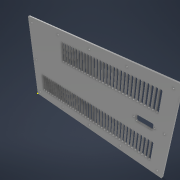
# Autodesk Inventor part: BackShield
Saved by Autodesk Inventor 2022 (Build 260153000, 153)
## iProperties
Created: 2022-04-28
Part Number: BackShield
Material: Типовые
Document SubType Name: Modeling
Designer: Kalugin_a
Density: 1 g/cm^3
Appearance: Анодированный — светло-серый
Author: Kalugin_a
Autodesk Inventor part; units mm, degrees
ref_plane "YZ Plane" through (0, 0, 0) normal (1, 0, 0) x (0, 1, 0)
ref_plane "XZ Plane" through (0, 0, 0) normal (0, 1, 0) x (-1, 0, 0)
ref_plane "XY Plane" through (0, 0, 0) normal (0, 0, 1) x (1, 0, 0)
ref_plane "РабПлоскость5" through (0, 0, 0) normal (0, 0, 1) x (1, 0, 0)
sketch "Эскиз1" plane through (0, 0, 0) normal (0, 0, 1) x (1, 0, 0)
  line L0 (2, 0) -> (280, 0)
  line L1 (282, 2) -> (282, 154)
  line L2 (280, 156) -> (2, 156)
  line L3 (0, 154) -> (0, 2)
  arc A0 (282, 154) -> (280, 156) centre (280, 154) ccw
  arc A1 (280, 0) -> (282, 2) centre (280, 2) ccw
  arc A2 (2, 156) -> (0, 154) centre (2, 154) ccw
  arc A3 (0, 2) -> (2, 0) centre (2, 2) ccw
  line L4 (264, 18) -> (18, 18) construction
  line L5 (9, 147) -> (273, 147) construction
  line L6 (273, 147) -> (273, 9) construction
  line L7 (273, 9) -> (9, 9) construction
  line L8 (9, 9) -> (9, 147) construction
  line L9 (24, 54.125) -> (24, 54.125)
  line L10 (26, 52.125) -> (26, 21.125)
  line L11 (24, 19.125) -> (24, 19.125)
  line L12 (22, 21.125) -> (22, 52.125)
  arc A4 (22, 21.125) -> (24, 19.125) centre (24, 21.125) ccw
  arc A5 (24, 19.125) -> (26, 21.125) centre (24, 21.125) ccw
  arc A6 (24, 54.125) -> (22, 52.125) centre (24, 52.125) ccw
  arc A7 (26, 52.125) -> (24, 54.125) centre (24, 52.125) ccw
  line L13 (30, 19.125) -> (30, 19.125)
  arc A8 (30, 19.125) -> (32, 21.125) centre (30, 21.125) ccw
  line L14 (32, 52.125) -> (32, 21.125)
  arc A9 (32, 52.125) -> (30, 54.125) centre (30, 52.125) ccw
  line L15 (30, 54.125) -> (30, 54.125)
  arc A10 (30, 54.125) -> (28, 52.125) centre (30, 52.125) ccw
  line L16 (28, 21.125) -> (28, 52.125)
  arc A11 (28, 21.125) -> (30, 19.125) centre (30, 21.125) ccw
  line L17 (36, 19.125) -> (36, 19.125)
  arc A12 (36, 19.125) -> (38, 21.125) centre (36, 21.125) ccw
  line L18 (38, 52.125) -> (38, 21.125)
  arc A13 (38, 52.125) -> (36, 54.125) centre (36, 52.125) ccw
  line L19 (36, 54.125) -> (36, 54.125)
  arc A14 (36, 54.125) -> (34, 52.125) centre (36, 52.125) ccw
  line L20 (34, 21.125) -> (34, 52.125)
  arc A15 (34, 21.125) -> (36, 19.125) centre (36, 21.125) ccw
  line L21 (42, 19.125) -> (42, 19.125)
  arc A16 (42, 19.125) -> (44, 21.125) centre (42, 21.125) ccw
  line L22 (44, 52.125) -> (44, 21.125)
  arc A17 (44, 52.125) -> (42, 54.125) centre (42, 52.125) ccw
  line L23 (42, 54.125) -> (42, 54.125)
  arc A18 (42, 54.125) -> (40, 52.125) centre (42, 52.125) ccw
  line L24 (40, 21.125) -> (40, 52.125)
  arc A19 (40, 21.125) -> (42, 19.125) centre (42, 21.125) ccw
  line L25 (48, 19.125) -> (48, 19.125)
  arc A20 (48, 19.125) -> (50, 21.125) centre (48, 21.125) ccw
  line L26 (50, 52.125) -> (50, 21.125)
  arc A21 (50, 52.125) -> (48, 54.125) centre (48, 52.125) ccw
  line L27 (48, 54.125) -> (48, 54.125)
  arc A22 (48, 54.125) -> (46, 52.125) centre (48, 52.125) ccw
  line L28 (46, 21.125) -> (46, 52.125)
  arc A23 (46, 21.125) -> (48, 19.125) centre (48, 21.125) ccw
  line L29 (54, 19.125) -> (54, 19.125)
  arc A24 (54, 19.125) -> (56, 21.125) centre (54, 21.125) ccw
  line L30 (56, 52.125) -> (56, 21.125)
  arc A25 (56, 52.125) -> (54, 54.125) centre (54, 52.125) ccw
  line L31 (54, 54.125) -> (54, 54.125)
  arc A26 (54, 54.125) -> (52, 52.125) centre (54, 52.125) ccw
  line L32 (52, 21.125) -> (52, 52.125)
  arc A27 (52, 21.125) -> (54, 19.125) centre (54, 21.125) ccw
  line L33 (60, 19.125) -> (60, 19.125)
  arc A28 (60, 19.125) -> (62, 21.125) centre (60, 21.125) ccw
  line L34 (62, 52.125) -> (62, 21.125)
  arc A29 (62, 52.125) -> (60, 54.125) centre (60, 52.125) ccw
  line L35 (60, 54.125) -> (60, 54.125)
  arc A30 (60, 54.125) -> (58, 52.125) centre (60, 52.125) ccw
  line L36 (58, 21.125) -> (58, 52.125)
  arc A31 (58, 21.125) -> (60, 19.125) centre (60, 21.125) ccw
  line L37 (66, 19.125) -> (66, 19.125)
  arc A32 (66, 19.125) -> (68, 21.125) centre (66, 21.125) ccw
  line L38 (68, 52.125) -> (68, 21.125)
  arc A33 (68, 52.125) -> (66, 54.125) centre (66, 52.125) ccw
  line L39 (66, 54.125) -> (66, 54.125)
  arc A34 (66, 54.125) -> (64, 52.125) centre (66, 52.125) ccw
  line L40 (64, 21.125) -> (64, 52.125)
  arc A35 (64, 21.125) -> (66, 19.125) centre (66, 21.125) ccw
  line L41 (72, 19.125) -> (72, 19.125)
  arc A36 (72, 19.125) -> (74, 21.125) centre (72, 21.125) ccw
  line L42 (74, 52.125) -> (74, 21.125)
  arc A37 (74, 52.125) -> (72, 54.125) centre (72, 52.125) ccw
  line L43 (72, 54.125) -> (72, 54.125)
  arc A38 (72, 54.125) -> (70, 52.125) centre (72, 52.125) ccw
  line L44 (70, 21.125) -> (70, 52.125)
  arc A39 (70, 21.125) -> (72, 19.125) centre (72, 21.125) ccw
  line L45 (78, 19.125) -> (78, 19.125)
  arc A40 (78, 19.125) -> (80, 21.125) centre (78, 21.125) ccw
  line L46 (80, 52.125) -> (80, 21.125)
  arc A41 (80, 52.125) -> (78, 54.125) centre (78, 52.125) ccw
  line L47 (78, 54.125) -> (78, 54.125)
  arc A42 (78, 54.125) -> (76, 52.125) centre (78, 52.125) ccw
  line L48 (76, 21.125) -> (76, 52.125)
  arc A43 (76, 21.125) -> (78, 19.125) centre (78, 21.125) ccw
  line L49 (84, 19.125) -> (84, 19.125)
  arc A44 (84, 19.125) -> (86, 21.125) centre (84, 21.125) ccw
  line L50 (86, 52.125) -> (86, 21.125)
  arc A45 (86, 52.125) -> (84, 54.125) centre (84, 52.125) ccw
  line L51 (84, 54.125) -> (84, 54.125)
  arc A46 (84, 54.125) -> (82, 52.125) centre (84, 52.125) ccw
  line L52 (82, 21.125) -> (82, 52.125)
  arc A47 (82, 21.125) -> (84, 19.125) centre (84, 21.125) ccw
  line L53 (90, 19.125) -> (90, 19.125)
  arc A48 (90, 19.125) -> (92, 21.125) centre (90, 21.125) ccw
  line L54 (92, 52.125) -> (92, 21.125)
  arc A49 (92, 52.125) -> (90, 54.125) centre (90, 52.125) ccw
  line L55 (90, 54.125) -> (90, 54.125)
  arc A50 (90, 54.125) -> (88, 52.125) centre (90, 52.125) ccw
  line L56 (88, 21.125) -> (88, 52.125)
  arc A51 (88, 21.125) -> (90, 19.125) centre (90, 21.125) ccw
  line L57 (96, 19.125) -> (96, 19.125)
  arc A52 (96, 19.125) -> (98, 21.125) centre (96, 21.125) ccw
  line L58 (98, 52.125) -> (98, 21.125)
  arc A53 (98, 52.125) -> (96, 54.125) centre (96, 52.125) ccw
  line L59 (96, 54.125) -> (96, 54.125)
  arc A54 (96, 54.125) -> (94, 52.125) centre (96, 52.125) ccw
  line L60 (94, 21.125) -> (94, 52.125)
  arc A55 (94, 21.125) -> (96, 19.125) centre (96, 21.125) ccw
  line L61 (102, 19.125) -> (102, 19.125)
  arc A56 (102, 19.125) -> (104, 21.125) centre (102, 21.125) ccw
  line L62 (104, 52.125) -> (104, 21.125)
  arc A57 (104, 52.125) -> (102, 54.125) centre (102, 52.125) ccw
  line L63 (102, 54.125) -> (102, 54.125)
  arc A58 (102, 54.125) -> (100, 52.125) centre (102, 52.125) ccw
  line L64 (100, 21.125) -> (100, 52.125)
  arc A59 (100, 21.125) -> (102, 19.125) centre (102, 21.125) ccw
  line L65 (108, 19.125) -> (108, 19.125)
  arc A60 (108, 19.125) -> (110, 21.125) centre (108, 21.125) ccw
  line L66 (110, 52.125) -> (110, 21.125)
  arc A61 (110, 52.125) -> (108, 54.125) centre (108, 52.125) ccw
  line L67 (108, 54.125) -> (108, 54.125)
  arc A62 (108, 54.125) -> (106, 52.125) centre (108, 52.125) ccw
  line L68 (106, 21.125) -> (106, 52.125)
  arc A63 (106, 21.125) -> (108, 19.125) centre (108, 21.125) ccw
  line L69 (114, 19.125) -> (114, 19.125)
  arc A64 (114, 19.125) -> (116, 21.125) centre (114, 21.125) ccw
  line L70 (116, 52.125) -> (116, 21.125)
  arc A65 (116, 52.125) -> (114, 54.125) centre (114, 52.125) ccw
  line L71 (114, 54.125) -> (114, 54.125)
  arc A66 (114, 54.125) -> (112, 52.125) centre (114, 52.125) ccw
  line L72 (112, 21.125) -> (112, 52.125)
  arc A67 (112, 21.125) -> (114, 19.125) centre (114, 21.125) ccw
  line L73 (120, 19.125) -> (120, 19.125)
  arc A68 (120, 19.125) -> (122, 21.125) centre (120, 21.125) ccw
  line L74 (122, 52.125) -> (122, 21.125)
  arc A69 (122, 52.125) -> (120, 54.125) centre (120, 52.125) ccw
  line L75 (120, 54.125) -> (120, 54.125)
  arc A70 (120, 54.125) -> (118, 52.125) centre (120, 52.125) ccw
  line L76 (118, 21.125) -> (118, 52.125)
  arc A71 (118, 21.125) -> (120, 19.125) centre (120, 21.125) ccw
  line L77 (126, 19.125) -> (126, 19.125)
  arc A72 (126, 19.125) -> (128, 21.125) centre (126, 21.125) ccw
  line L78 (128, 52.125) -> (128, 21.125)
  arc A73 (128, 52.125) -> (126, 54.125) centre (126, 52.125) ccw
  line L79 (126, 54.125) -> (126, 54.125)
  arc A74 (126, 54.125) -> (124, 52.125) centre (126, 52.125) ccw
  line L80 (124, 21.125) -> (124, 52.125)
  arc A75 (124, 21.125) -> (126, 19.125) centre (126, 21.125) ccw
  line L81 (132, 19.125) -> (132, 19.125)
  arc A76 (132, 19.125) -> (134, 21.125) centre (132, 21.125) ccw
  line L82 (134, 52.125) -> (134, 21.125)
  arc A77 (134, 52.125) -> (132, 54.125) centre (132, 52.125) ccw
  line L83 (132, 54.125) -> (132, 54.125)
  arc A78 (132, 54.125) -> (130, 52.125) centre (132, 52.125) ccw
  line L84 (130, 21.125) -> (130, 52.125)
  arc A79 (130, 21.125) -> (132, 19.125) centre (132, 21.125) ccw
  line L85 (138, 19.125) -> (138, 19.125)
  arc A80 (138, 19.125) -> (140, 21.125) centre (138, 21.125) ccw
  line L86 (140, 52.125) -> (140, 21.125)
  arc A81 (140, 52.125) -> (138, 54.125) centre (138, 52.125) ccw
  line L87 (138, 54.125) -> (138, 54.125)
  arc A82 (138, 54.125) -> (136, 52.125) centre (138, 52.125) ccw
  line L88 (136, 21.125) -> (136, 52.125)
  arc A83 (136, 21.125) -> (138, 19.125) centre (138, 21.125) ccw
  line L89 (144, 19.125) -> (144, 19.125)
  arc A84 (144, 19.125) -> (146, 21.125) centre (144, 21.125) ccw
  line L90 (146, 52.125) -> (146, 21.125)
  arc A85 (146, 52.125) -> (144, 54.125) centre (144, 52.125) ccw
  line L91 (144, 54.125) -> (144, 54.125)
  arc A86 (144, 54.125) -> (142, 52.125) centre (144, 52.125) ccw
  line L92 (142, 21.125) -> (142, 52.125)
  arc A87 (142, 21.125) -> (144, 19.125) centre (144, 21.125) ccw
  line L93 (150, 19.125) -> (150, 19.125)
  arc A88 (150, 19.125) -> (152, 21.125) centre (150, 21.125) ccw
  line L94 (152, 52.125) -> (152, 21.125)
  arc A89 (152, 52.125) -> (150, 54.125) centre (150, 52.125) ccw
  line L95 (150, 54.125) -> (150, 54.125)
  arc A90 (150, 54.125) -> (148, 52.125) centre (150, 52.125) ccw
  line L96 (148, 21.125) -> (148, 52.125)
  arc A91 (148, 21.125) -> (150, 19.125) centre (150, 21.125) ccw
  line L97 (156, 19.125) -> (156, 19.125)
  arc A92 (156, 19.125) -> (158, 21.125) centre (156, 21.125) ccw
  line L98 (158, 52.125) -> (158, 21.125)
  arc A93 (158, 52.125) -> (156, 54.125) centre (156, 52.125) ccw
  line L99 (156, 54.125) -> (156, 54.125)
  arc A94 (156, 54.125) -> (154, 52.125) centre (156, 52.125) ccw
  line L100 (154, 21.125) -> (154, 52.125)
  arc A95 (154, 21.125) -> (156, 19.125) centre (156, 21.125) ccw
  line L101 (162, 19.125) -> (162, 19.125)
  arc A96 (162, 19.125) -> (164, 21.125) centre (162, 21.125) ccw
  line L102 (164, 52.125) -> (164, 21.125)
  arc A97 (164, 52.125) -> (162, 54.125) centre (162, 52.125) ccw
  line L103 (162, 54.125) -> (162, 54.125)
  arc A98 (162, 54.125) -> (160, 52.125) centre (162, 52.125) ccw
  line L104 (160, 21.125) -> (160, 52.125)
  arc A99 (160, 21.125) -> (162, 19.125) centre (162, 21.125) ccw
  line L105 (168, 19.125) -> (168, 19.125)
  arc A100 (168, 19.125) -> (170, 21.125) centre (168, 21.125) ccw
  line L106 (170, 52.125) -> (170, 21.125)
  arc A101 (170, 52.125) -> (168, 54.125) centre (168, 52.125) ccw
  line L107 (168, 54.125) -> (168, 54.125)
  arc A102 (168, 54.125) -> (166, 52.125) centre (168, 52.125) ccw
  line L108 (166, 21.125) -> (166, 52.125)
  arc A103 (166, 21.125) -> (168, 19.125) centre (168, 21.125) ccw
  line L109 (174, 19.125) -> (174, 19.125)
  arc A104 (174, 19.125) -> (176, 21.125) centre (174, 21.125) ccw
  line L110 (176, 52.125) -> (176, 21.125)
  arc A105 (176, 52.125) -> (174, 54.125) centre (174, 52.125) ccw
  line L111 (174, 54.125) -> (174, 54.125)
  arc A106 (174, 54.125) -> (172, 52.125) centre (174, 52.125) ccw
  line L112 (172, 21.125) -> (172, 52.125)
  arc A107 (172, 21.125) -> (174, 19.125) centre (174, 21.125) ccw
  line L113 (180, 19.125) -> (180, 19.125)
  arc A108 (180, 19.125) -> (182, 21.125) centre (180, 21.125) ccw
  line L114 (182, 52.125) -> (182, 21.125)
  arc A109 (182, 52.125) -> (180, 54.125) centre (180, 52.125) ccw
  line L115 (180, 54.125) -> (180, 54.125)
  arc A110 (180, 54.125) -> (178, 52.125) centre (180, 52.125) ccw
  line L116 (178, 21.125) -> (178, 52.125)
  arc A111 (178, 21.125) -> (180, 19.125) centre (180, 21.125) ccw
  line L117 (186, 19.125) -> (186, 19.125)
  arc A112 (186, 19.125) -> (188, 21.125) centre (186, 21.125) ccw
  line L118 (188, 52.125) -> (188, 21.125)
  arc A113 (188, 52.125) -> (186, 54.125) centre (186, 52.125) ccw
  line L119 (186, 54.125) -> (186, 54.125)
  arc A114 (186, 54.125) -> (184, 52.125) centre (186, 52.125) ccw
  line L120 (184, 21.125) -> (184, 52.125)
  arc A115 (184, 21.125) -> (186, 19.125) centre (186, 21.125) ccw
  line L121 (192, 19.125) -> (192, 19.125)
  arc A116 (192, 19.125) -> (194, 21.125) centre (192, 21.125) ccw
  line L122 (194, 52.125) -> (194, 21.125)
  arc A117 (194, 52.125) -> (192, 54.125) centre (192, 52.125) ccw
  line L123 (192, 54.125) -> (192, 54.125)
  arc A118 (192, 54.125) -> (190, 52.125) centre (192, 52.125) ccw
  line L124 (190, 21.125) -> (190, 52.125)
  arc A119 (190, 21.125) -> (192, 19.125) centre (192, 21.125) ccw
  line L125 (198, 19.125) -> (198, 19.125)
  arc A120 (198, 19.125) -> (200, 21.125) centre (198, 21.125) ccw
  line L126 (200, 52.125) -> (200, 21.125)
  arc A121 (200, 52.125) -> (198, 54.125) centre (198, 52.125) ccw
  line L127 (198, 54.125) -> (198, 54.125)
  arc A122 (198, 54.125) -> (196, 52.125) centre (198, 52.125) ccw
  line L128 (196, 21.125) -> (196, 52.125)
  arc A123 (196, 21.125) -> (198, 19.125) centre (198, 21.125) ccw
  line L129 (204, 19.125) -> (204, 19.125)
  arc A124 (204, 19.125) -> (206, 21.125) centre (204, 21.125) ccw
  line L130 (206, 52.125) -> (206, 21.125)
  arc A125 (206, 52.125) -> (204, 54.125) centre (204, 52.125) ccw
  line L131 (204, 54.125) -> (204, 54.125)
  arc A126 (204, 54.125) -> (202, 52.125) centre (204, 52.125) ccw
  line L132 (202, 21.125) -> (202, 52.125)
  arc A127 (202, 21.125) -> (204, 19.125) centre (204, 21.125) ccw
  line L133 (210, 19.125) -> (210, 19.125)
  arc A128 (210, 19.125) -> (212, 21.125) centre (210, 21.125) ccw
  line L134 (212, 52.125) -> (212, 21.125)
  arc A129 (212, 52.125) -> (210, 54.125) centre (210, 52.125) ccw
  line L135 (210, 54.125) -> (210, 54.125)
  arc A130 (210, 54.125) -> (208, 52.125) centre (210, 52.125) ccw
  line L136 (208, 21.125) -> (208, 52.125)
  arc A131 (208, 21.125) -> (210, 19.125) centre (210, 21.125) ccw
  line L137 (216, 19.125) -> (216, 19.125)
  arc A132 (216, 19.125) -> (218, 21.125) centre (216, 21.125) ccw
  line L138 (218, 52.125) -> (218, 21.125)
  arc A133 (218, 52.125) -> (216, 54.125) centre (216, 52.125) ccw
  line L139 (216, 54.125) -> (216, 54.125)
  arc A134 (216, 54.125) -> (214, 52.125) centre (216, 52.125) ccw
  line L140 (214, 21.125) -> (214, 52.125)
  arc A135 (214, 21.125) -> (216, 19.125) centre (216, 21.125) ccw
  line L141 (222, 19.125) -> (222, 19.125)
  arc A136 (222, 19.125) -> (224, 21.125) centre (222, 21.125) ccw
  line L142 (224, 52.125) -> (224, 21.125)
  arc A137 (224, 52.125) -> (222, 54.125) centre (222, 52.125) ccw
  line L143 (222, 54.125) -> (222, 54.125)
  arc A138 (222, 54.125) -> (220, 52.125) centre (222, 52.125) ccw
  line L144 (220, 21.125) -> (220, 52.125)
  arc A139 (220, 21.125) -> (222, 19.125) centre (222, 21.125) ccw
  line L145 (228, 19.125) -> (228, 19.125)
  arc A140 (228, 19.125) -> (230, 21.125) centre (228, 21.125) ccw
  line L146 (230, 52.125) -> (230, 21.125)
  arc A141 (230, 52.125) -> (228, 54.125) centre (228, 52.125) ccw
  line L147 (228, 54.125) -> (228, 54.125)
  arc A142 (228, 54.125) -> (226, 52.125) centre (228, 52.125) ccw
  line L148 (226, 21.125) -> (226, 52.125)
  arc A143 (226, 21.125) -> (228, 19.125) centre (228, 21.125) ccw
  line L149 (234, 19.125) -> (234, 19.125)
  arc A144 (234, 19.125) -> (236, 21.125) centre (234, 21.125) ccw
  line L150 (236, 52.125) -> (236, 21.125)
  arc A145 (236, 52.125) -> (234, 54.125) centre (234, 52.125) ccw
  line L151 (234, 54.125) -> (234, 54.125)
  arc A146 (234, 54.125) -> (232, 52.125) centre (234, 52.125) ccw
  line L152 (232, 21.125) -> (232, 52.125)
  arc A147 (232, 21.125) -> (234, 19.125) centre (234, 21.125) ccw
  line L153 (240, 19.125) -> (240, 19.125)
  arc A148 (240, 19.125) -> (242, 21.125) centre (240, 21.125) ccw
  line L154 (242, 52.125) -> (242, 21.125)
  arc A149 (242, 52.125) -> (240, 54.125) centre (240, 52.125) ccw
  line L155 (240, 54.125) -> (240, 54.125)
  arc A150 (240, 54.125) -> (238, 52.125) centre (240, 52.125) ccw
  line L156 (238, 21.125) -> (238, 52.125)
  arc A151 (238, 21.125) -> (240, 19.125) centre (240, 21.125) ccw
  line L157 (246, 19.125) -> (246, 19.125)
  arc A152 (246, 19.125) -> (248, 21.125) centre (246, 21.125) ccw
  line L158 (248, 52.125) -> (248, 21.125)
  arc A153 (248, 52.125) -> (246, 54.125) centre (246, 52.125) ccw
  line L159 (246, 54.125) -> (246, 54.125)
  arc A154 (246, 54.125) -> (244, 52.125) centre (246, 52.125) ccw
  line L160 (244, 21.125) -> (244, 52.125)
  arc A155 (244, 21.125) -> (246, 19.125) centre (246, 21.125) ccw
  line L161 (252, 19.125) -> (252, 19.125)
  arc A156 (252, 19.125) -> (254, 21.125) centre (252, 21.125) ccw
  line L162 (254, 52.125) -> (254, 21.125)
  arc A157 (254, 52.125) -> (252, 54.125) centre (252, 52.125) ccw
  line L163 (252, 54.125) -> (252, 54.125)
  arc A158 (252, 54.125) -> (250, 52.125) centre (252, 52.125) ccw
  line L164 (250, 21.125) -> (250, 52.125)
  arc A159 (250, 21.125) -> (252, 19.125) centre (252, 21.125) ccw
  line L165 (258, 19.125) -> (258, 19.125)
  arc A160 (258, 19.125) -> (260, 21.125) centre (258, 21.125) ccw
  line L166 (260, 52.125) -> (260, 21.125)
  arc A161 (260, 52.125) -> (258, 54.125) centre (258, 52.125) ccw
  line L167 (258, 54.125) -> (258, 54.125)
  arc A162 (258, 54.125) -> (256, 52.125) centre (258, 52.125) ccw
  line L168 (256, 21.125) -> (256, 52.125)
  arc A163 (256, 21.125) -> (258, 19.125) centre (258, 21.125) ccw
  line L169 (86, 136) -> (86, 105)
  line L170 (82, 105) -> (82, 136)
  arc A164 (84, 138) -> (82, 136) centre (84, 136) ccw
  arc A165 (86, 136) -> (84, 138) centre (84, 136) ccw
  arc A166 (82, 105) -> (84, 103) centre (84, 105) ccw
  arc A167 (84, 103) -> (86, 105) centre (84, 105) ccw
  arc A168 (90, 103) -> (92, 105) centre (90, 105) ccw
  arc A169 (88, 105) -> (90, 103) centre (90, 105) ccw
  line L171 (92, 136) -> (92, 105)
  line L172 (88, 105) -> (88, 136)
  arc A170 (92, 136) -> (90, 138) centre (90, 136) ccw
  arc A171 (90, 138) -> (88, 136) centre (90, 136) ccw
  arc A172 (96, 103) -> (98, 105) centre (96, 105) ccw
  arc A173 (94, 105) -> (96, 103) centre (96, 105) ccw
  line L173 (98, 136) -> (98, 105)
  line L174 (94, 105) -> (94, 136)
  arc A174 (98, 136) -> (96, 138) centre (96, 136) ccw
  arc A175 (96, 138) -> (94, 136) centre (96, 136) ccw
  arc A176 (102, 103) -> (104, 105) centre (102, 105) ccw
  arc A177 (100, 105) -> (102, 103) centre (102, 105) ccw
  line L175 (104, 136) -> (104, 105)
  line L176 (100, 105) -> (100, 136)
  arc A178 (104, 136) -> (102, 138) centre (102, 136) ccw
  arc A179 (102, 138) -> (100, 136) centre (102, 136) ccw
  arc A180 (108, 103) -> (110, 105) centre (108, 105) ccw
  arc A181 (106, 105) -> (108, 103) centre (108, 105) ccw
  line L177 (110, 136) -> (110, 105)
  line L178 (106, 105) -> (106, 136)
  arc A182 (110, 136) -> (108, 138) centre (108, 136) ccw
  arc A183 (108, 138) -> (106, 136) centre (108, 136) ccw
  arc A184 (114, 103) -> (116, 105) centre (114, 105) ccw
  arc A185 (112, 105) -> (114, 103) centre (114, 105) ccw
  line L179 (116, 136) -> (116, 105)
  line L180 (112, 105) -> (112, 136)
  arc A186 (116, 136) -> (114, 138) centre (114, 136) ccw
  arc A187 (114, 138) -> (112, 136) centre (114, 136) ccw
  arc A188 (120, 103) -> (122, 105) centre (120, 105) ccw
  arc A189 (118, 105) -> (120, 103) centre (120, 105) ccw
  line L181 (122, 136) -> (122, 105)
  line L182 (118, 105) -> (118, 136)
  arc A190 (122, 136) -> (120, 138) centre (120, 136) ccw
  arc A191 (120, 138) -> (118, 136) centre (120, 136) ccw
  arc A192 (126, 103) -> (128, 105) centre (126, 105) ccw
  arc A193 (124, 105) -> (126, 103) centre (126, 105) ccw
  line L183 (128, 136) -> (128, 105)
  line L184 (124, 105) -> (124, 136)
  arc A194 (128, 136) -> (126, 138) centre (126, 136) ccw
  arc A195 (126, 138) -> (124, 136) centre (126, 136) ccw
  arc A196 (132, 103) -> (134, 105) centre (132, 105) ccw
  arc A197 (130, 105) -> (132, 103) centre (132, 105) ccw
  line L185 (134, 136) -> (134, 105)
  line L186 (130, 105) -> (130, 136)
  arc A198 (134, 136) -> (132, 138) centre (132, 136) ccw
  arc A199 (132, 138) -> (130, 136) centre (132, 136) ccw
  arc A200 (138, 103) -> (140, 105) centre (138, 105) ccw
  arc A201 (136, 105) -> (138, 103) centre (138, 105) ccw
  line L187 (140, 136) -> (140, 105)
  line L188 (136, 105) -> (136, 136)
  arc A202 (140, 136) -> (138, 138) centre (138, 136) ccw
  arc A203 (138, 138) -> (136, 136) centre (138, 136) ccw
  arc A204 (144, 103) -> (146, 105) centre (144, 105) ccw
  arc A205 (142, 105) -> (144, 103) centre (144, 105) ccw
  line L189 (146, 136) -> (146, 105)
  line L190 (142, 105) -> (142, 136)
  arc A206 (146, 136) -> (144, 138) centre (144, 136) ccw
  arc A207 (144, 138) -> (142, 136) centre (144, 136) ccw
  arc A208 (150, 103) -> (152, 105) centre (150, 105) ccw
  arc A209 (148, 105) -> (150, 103) centre (150, 105) ccw
  line L191 (152, 136) -> (152, 105)
  line L192 (148, 105) -> (148, 136)
  arc A210 (152, 136) -> (150, 138) centre (150, 136) ccw
  arc A211 (150, 138) -> (148, 136) centre (150, 136) ccw
  arc A212 (156, 103) -> (158, 105) centre (156, 105) ccw
  arc A213 (154, 105) -> (156, 103) centre (156, 105) ccw
  line L193 (158, 136) -> (158, 105)
  line L194 (154, 105) -> (154, 136)
  arc A214 (158, 136) -> (156, 138) centre (156, 136) ccw
  arc A215 (156, 138) -> (154, 136) centre (156, 136) ccw
  arc A216 (162, 103) -> (164, 105) centre (162, 105) ccw
  arc A217 (160, 105) -> (162, 103) centre (162, 105) ccw
  line L195 (164, 136) -> (164, 105)
  line L196 (160, 105) -> (160, 136)
  arc A218 (164, 136) -> (162, 138) centre (162, 136) ccw
  arc A219 (162, 138) -> (160, 136) centre (162, 136) ccw
  arc A220 (168, 103) -> (170, 105) centre (168, 105) ccw
  arc A221 (166, 105) -> (168, 103) centre (168, 105) ccw
  line L197 (170, 136) -> (170, 105)
  line L198 (166, 105) -> (166, 136)
  arc A222 (170, 136) -> (168, 138) centre (168, 136) ccw
  arc A223 (168, 138) -> (166, 136) centre (168, 136) ccw
  arc A224 (174, 103) -> (176, 105) centre (174, 105) ccw
  arc A225 (172, 105) -> (174, 103) centre (174, 105) ccw
  line L199 (176, 136) -> (176, 105)
  line L200 (172, 105) -> (172, 136)
  arc A226 (176, 136) -> (174, 138) centre (174, 136) ccw
  arc A227 (174, 138) -> (172, 136) centre (174, 136) ccw
  arc A228 (180, 103) -> (182, 105) centre (180, 105) ccw
  arc A229 (178, 105) -> (180, 103) centre (180, 105) ccw
  line L201 (182, 136) -> (182, 105)
  line L202 (178, 105) -> (178, 136)
  arc A230 (182, 136) -> (180, 138) centre (180, 136) ccw
  arc A231 (180, 138) -> (178, 136) centre (180, 136) ccw
  arc A232 (186, 103) -> (188, 105) centre (186, 105) ccw
  arc A233 (184, 105) -> (186, 103) centre (186, 105) ccw
  line L203 (188, 136) -> (188, 105)
  line L204 (184, 105) -> (184, 136)
  arc A234 (188, 136) -> (186, 138) centre (186, 136) ccw
  arc A235 (186, 138) -> (184, 136) centre (186, 136) ccw
  arc A236 (192, 103) -> (194, 105) centre (192, 105) ccw
  arc A237 (190, 105) -> (192, 103) centre (192, 105) ccw
  line L205 (194, 136) -> (194, 105)
  line L206 (190, 105) -> (190, 136)
  arc A238 (194, 136) -> (192, 138) centre (192, 136) ccw
  arc A239 (192, 138) -> (190, 136) centre (192, 136) ccw
  arc A240 (198, 103) -> (200, 105) centre (198, 105) ccw
  arc A241 (196, 105) -> (198, 103) centre (198, 105) ccw
  line L207 (200, 136) -> (200, 105)
  line L208 (196, 105) -> (196, 136)
  arc A242 (200, 136) -> (198, 138) centre (198, 136) ccw
  arc A243 (198, 138) -> (196, 136) centre (198, 136) ccw
  arc A244 (204, 103) -> (206, 105) centre (204, 105) ccw
  arc A245 (202, 105) -> (204, 103) centre (204, 105) ccw
  line L209 (206, 136) -> (206, 105)
  line L210 (202, 105) -> (202, 136)
  arc A246 (206, 136) -> (204, 138) centre (204, 136) ccw
  arc A247 (204, 138) -> (202, 136) centre (204, 136) ccw
  arc A248 (210, 103) -> (212, 105) centre (210, 105) ccw
  arc A249 (208, 105) -> (210, 103) centre (210, 105) ccw
  line L211 (212, 136) -> (212, 105)
  line L212 (208, 105) -> (208, 136)
  arc A250 (212, 136) -> (210, 138) centre (210, 136) ccw
  arc A251 (210, 138) -> (208, 136) centre (210, 136) ccw
  arc A252 (216, 103) -> (218, 105) centre (216, 105) ccw
  arc A253 (214, 105) -> (216, 103) centre (216, 105) ccw
  line L213 (218, 136) -> (218, 105)
  line L214 (214, 105) -> (214, 136)
  arc A254 (218, 136) -> (216, 138) centre (216, 136) ccw
  arc A255 (216, 138) -> (214, 136) centre (216, 136) ccw
  arc A256 (222, 103) -> (224, 105) centre (222, 105) ccw
  arc A257 (220, 105) -> (222, 103) centre (222, 105) ccw
  line L215 (224, 136) -> (224, 105)
  line L216 (220, 105) -> (220, 136)
  arc A258 (224, 136) -> (222, 138) centre (222, 136) ccw
  arc A259 (222, 138) -> (220, 136) centre (222, 136) ccw
  arc A260 (228, 103) -> (230, 105) centre (228, 105) ccw
  arc A261 (226, 105) -> (228, 103) centre (228, 105) ccw
  line L217 (230, 136) -> (230, 105)
  line L218 (226, 105) -> (226, 136)
  arc A262 (230, 136) -> (228, 138) centre (228, 136) ccw
  arc A263 (228, 138) -> (226, 136) centre (228, 136) ccw
  arc A264 (234, 103) -> (236, 105) centre (234, 105) ccw
  arc A265 (232, 105) -> (234, 103) centre (234, 105) ccw
  line L219 (236, 136) -> (236, 105)
  line L220 (232, 105) -> (232, 136)
  arc A266 (236, 136) -> (234, 138) centre (234, 136) ccw
  arc A267 (234, 138) -> (232, 136) centre (234, 136) ccw
  arc A268 (240, 103) -> (242, 105) centre (240, 105) ccw
  arc A269 (238, 105) -> (240, 103) centre (240, 105) ccw
  line L221 (242, 136) -> (242, 105)
  line L222 (238, 105) -> (238, 136)
  arc A270 (242, 136) -> (240, 138) centre (240, 136) ccw
  arc A271 (240, 138) -> (238, 136) centre (240, 136) ccw
  arc A272 (246, 103) -> (248, 105) centre (246, 105) ccw
  arc A273 (244, 105) -> (246, 103) centre (246, 105) ccw
  line L223 (248, 136) -> (248, 105)
  line L224 (244, 105) -> (244, 136)
  arc A274 (248, 136) -> (246, 138) centre (246, 136) ccw
  arc A275 (246, 138) -> (244, 136) centre (246, 136) ccw
  arc A276 (252, 103) -> (254, 105) centre (252, 105) ccw
  arc A277 (250, 105) -> (252, 103) centre (252, 105) ccw
  line L225 (254, 136) -> (254, 105)
  line L226 (250, 105) -> (250, 136)
  arc A278 (254, 136) -> (252, 138) centre (252, 136) ccw
  arc A279 (252, 138) -> (250, 136) centre (252, 136) ccw
  arc A280 (258, 103) -> (260, 105) centre (258, 105) ccw
  arc A281 (256, 105) -> (258, 103) centre (258, 105) ccw
  line L227 (260, 136) -> (260, 105)
  line L228 (256, 105) -> (256, 136)
  arc A282 (260, 136) -> (258, 138) centre (258, 136) ccw
  arc A283 (258, 138) -> (256, 136) centre (258, 136) ccw
  line L229 (230.7241, 83.5644) -> (253.7241, 83.5644)
  line L230 (255.7241, 81.5644) -> (255.7241, 74.5644)
  line L231 (253.7241, 72.5644) -> (230.7241, 72.5644)
  line L232 (228.7241, 74.5644) -> (228.7241, 81.5644)
  circle A284 centre (258.6992, 78.0644) radius 1.5
  circle A285 centre (225.3792, 78.0644) radius 1.5
  arc A286 (230.7241, 83.5644) -> (228.7241, 81.5644) centre (230.7241, 81.5644) ccw
  arc A287 (255.7241, 81.5644) -> (253.7241, 83.5644) centre (253.7241, 81.5644) ccw
  arc A288 (253.7241, 72.5644) -> (255.7241, 74.5644) centre (253.7241, 74.5644) ccw
  arc A289 (228.7241, 74.5644) -> (230.7241, 72.5644) centre (230.7241, 74.5644) ccw
  circle A290 centre (9, 147) radius 1.5
  circle A291 centre (75, 147) radius 1.5
  circle A292 centre (141, 147) radius 1.5
  circle A293 centre (207, 147) radius 1.5
  circle A294 centre (273, 147) radius 1.5
  circle A295 centre (9, 78) radius 1.5
  circle A296 centre (9, 9) radius 1.5
  circle A297 centre (273, 78) radius 1.5
  circle A298 centre (273, 9) radius 1.5
  circle A299 centre (75, 9) radius 1.5
  line L233 (339, 9) -> (75, 9) construction
  circle A300 centre (141, 9) radius 1.5
  line L234 (405, 9) -> (141, 9) construction
  circle A301 centre (207, 9) radius 1.5
  line L235 (471, 9) -> (207, 9) construction
  line L236 (0, 154) -> (282.0247, 154) construction
  line L237 (282.0247, 154) -> (282.0247, -2.0407) construction
  line L238 (282.0247, -2.0407) -> (0, -2.0407) construction
  line L239 (0, -2.0407) -> (0, 154) construction
  point P0 (0, 0)
  point P1 (282, 156)
  point P2 (282, 0)
  point P3 (26, 19.125)
  point P4 (26, 54.125)
  point P5 (22, 19.125)
  point P6 (32, 19.125)
  point P7 (28, 19.125)
  point P8 (32, 54.125)
  point P9 (38, 19.125)
  point P10 (34, 19.125)
  point P11 (38, 54.125)
  point P12 (44, 19.125)
  point P13 (40, 19.125)
  point P14 (44, 54.125)
  point P15 (50, 19.125)
  point P16 (46, 19.125)
  point P17 (50, 54.125)
  point P18 (56, 19.125)
  point P19 (52, 19.125)
  point P20 (56, 54.125)
  point P21 (62, 19.125)
  point P22 (58, 19.125)
  point P23 (62, 54.125)
  point P24 (68, 19.125)
  point P25 (64, 19.125)
  point P26 (68, 54.125)
  point P27 (74, 19.125)
  point P28 (70, 19.125)
  point P29 (74, 54.125)
  point P30 (80, 19.125)
  point P31 (76, 19.125)
  point P32 (80, 54.125)
  point P33 (86, 19.125)
  point P34 (82, 19.125)
  point P35 (86, 54.125)
  point P36 (92, 19.125)
  point P37 (88, 19.125)
  point P38 (92, 54.125)
  point P39 (98, 19.125)
  point P40 (94, 19.125)
  point P41 (98, 54.125)
  point P42 (104, 19.125)
  point P43 (100, 19.125)
  point P44 (104, 54.125)
  point P45 (110, 19.125)
  point P46 (106, 19.125)
  point P47 (110, 54.125)
  point P48 (116, 19.125)
  point P49 (112, 19.125)
  point P50 (116, 54.125)
  point P51 (122, 19.125)
  point P52 (118, 19.125)
  point P53 (122, 54.125)
  point P54 (128, 19.125)
  point P55 (124, 19.125)
  point P56 (128, 54.125)
  point P57 (134, 19.125)
  point P58 (130, 19.125)
  point P59 (134, 54.125)
  point P60 (140, 19.125)
  point P61 (136, 19.125)
  point P62 (140, 54.125)
  point P63 (146, 19.125)
  point P64 (142, 19.125)
  point P65 (146, 54.125)
  point P66 (152, 19.125)
  point P67 (148, 19.125)
  point P68 (152, 54.125)
  point P69 (158, 19.125)
  point P70 (154, 19.125)
  point P71 (158, 54.125)
  point P72 (164, 19.125)
  point P73 (160, 19.125)
  point P74 (164, 54.125)
  point P75 (170, 19.125)
  point P76 (166, 19.125)
  point P77 (170, 54.125)
  point P78 (176, 19.125)
  point P79 (172, 19.125)
  point P80 (176, 54.125)
  point P81 (182, 19.125)
  point P82 (178, 19.125)
  point P83 (182, 54.125)
  point P84 (188, 19.125)
  point P85 (184, 19.125)
  point P86 (188, 54.125)
  point P87 (194, 19.125)
  point P88 (190, 19.125)
  point P89 (194, 54.125)
  point P90 (200, 19.125)
  point P91 (196, 19.125)
  point P92 (200, 54.125)
  point P93 (206, 19.125)
  point P94 (202, 19.125)
  point P95 (206, 54.125)
  point P96 (212, 19.125)
  point P97 (208, 19.125)
  point P98 (212, 54.125)
  point P99 (218, 19.125)
  point P100 (214, 19.125)
  point P101 (218, 54.125)
  point P102 (224, 19.125)
  point P103 (220, 19.125)
  point P104 (224, 54.125)
  point P105 (230, 19.125)
  point P106 (226, 19.125)
  point P107 (230, 54.125)
  point P108 (236, 19.125)
  point P109 (232, 19.125)
  point P110 (236, 54.125)
  point P111 (242, 19.125)
  point P112 (238, 19.125)
  point P113 (242, 54.125)
  point P114 (248, 19.125)
  point P115 (244, 19.125)
  point P116 (248, 54.125)
  point P117 (254, 19.125)
  point P118 (250, 19.125)
  point P119 (254, 54.125)
  point P120 (260, 19.125)
  point P121 (256, 19.125)
  point P122 (260, 54.125)
  point P123 (86, 103)
  point P124 (86, 138)
  point P125 (82, 103)
  point P126 (92, 103)
  point P127 (88, 103)
  point P128 (92, 138)
  point P129 (98, 103)
  point P130 (94, 103)
  point P131 (98, 138)
  point P132 (104, 103)
  point P133 (100, 103)
  point P134 (104, 138)
  point P135 (110, 103)
  point P136 (106, 103)
  point P137 (110, 138)
  point P138 (116, 103)
  point P139 (112, 103)
  point P140 (116, 138)
  point P141 (122, 103)
  point P142 (118, 103)
  point P143 (122, 138)
  point P144 (128, 103)
  point P145 (124, 103)
  point P146 (128, 138)
  point P147 (134, 103)
  point P148 (130, 103)
  point P149 (134, 138)
  point P150 (140, 103)
  point P151 (136, 103)
  point P152 (140, 138)
  point P153 (146, 103)
  point P154 (142, 103)
  point P155 (146, 138)
  point P156 (152, 103)
  point P157 (148, 103)
  point P158 (152, 138)
  point P159 (158, 103)
  point P160 (154, 103)
  point P161 (158, 138)
  point P162 (164, 103)
  point P163 (160, 103)
  point P164 (164, 138)
  point P165 (170, 103)
  point P166 (166, 103)
  point P167 (170, 138)
  point P168 (176, 103)
  point P169 (172, 103)
  point P170 (176, 138)
  point P171 (182, 103)
  point P172 (178, 103)
  point P173 (182, 138)
  point P174 (188, 103)
  point P175 (184, 103)
  point P176 (188, 138)
  point P177 (194, 103)
  point P178 (190, 103)
  point P179 (194, 138)
  point P180 (200, 103)
  point P181 (196, 103)
  point P182 (200, 138)
  point P183 (206, 103)
  point P184 (202, 103)
  point P185 (206, 138)
  point P186 (212, 103)
  point P187 (208, 103)
  point P188 (212, 138)
  point P189 (218, 103)
  point P190 (214, 103)
  point P191 (218, 138)
  point P192 (224, 103)
  point P193 (220, 103)
  point P194 (224, 138)
  point P195 (230, 103)
  point P196 (226, 103)
  point P197 (230, 138)
  point P198 (236, 103)
  point P199 (232, 103)
  dimension "d1" = 156
  dimension "d2" = 2
  dimension "d7" = 264
  dimension "d8" = 138
  dimension "d9" = 9
  dimension "d10" = 9
  dimension "d11" = 4
  dimension "d12" = 35
  dimension "d13" = 2
  dimension "d16" = 6
  dimension "d21" = 22
  dimension "d30" = 6
  dimension "d35" = 27
  dimension "d36" = 11
  dimension "d38" = 3
  dimension "d39" = 33.32
  dimension "d40" = 2
  dimension "d43" = 3
  dimension "d46" = 66
  dimension "d53" = 69
  dimension "d60" = 69
  dimension "d67" = 66
  dimension "d76" = 82
  dimension "d77" = 2
  dimension "d92" = 282
  constraints: 576 point on circle, 472 end point, 342 point on line, 302 centre point, 36 horizontal, 19 tangent, 9 equal radius, 7 parallel, 3 perpendicular, 2 vertical, 1 coincident, 1 collinear, 1690 other
  measures "d1" distance of point (282, 156) point (282, 0)
  measures "d2" radius of A0
  measures "d7" distance of L6.end L7.end
  measures "d8" distance of L5.end L6.end
  measures "d9" distance between parallel lines of L0 L7
  measures "d10" distance between parallel lines of L3 L8
  measures "d11" distance of point (26, 19.125) point (22, 19.125)
  measures "d12" distance of point (26, 54.125) point (26, 19.125)
  measures "d13" radius of A4
  measures "d16" distance of point (26, 19.125) point (32, 19.125)
  measures "d21" distance between parallel lines of L3 L12
  measures "d30" distance of point (86, 103) point (92, 103)
  measures "d35" distance of point (255.724, 72.564) point (228.724, 72.564)
  measures "d36" distance of point (255.724, 83.564) point (255.724, 72.564)
  measures "d38" diameter of A285
  measures "d39" distance of A284.centre A285.centre
  measures "d40" radius of A286
  measures "d43" diameter of A290
  measures "d46" distance of A290.centre A291.centre
  measures "d53" distance of A290.centre A295.centre
  measures "d60" distance of A294.centre A297.centre
  measures "d67" distance of A296.centre A299.centre
  measures "d76" distance between parallel lines of L3 L170
  measures "d77" distance between parallel lines of L16 L10
  measures "d92" distance between parallel lines of L1 L3
extrude "Выдавливание2" add sketch "Эскиз1" along normal blind 3
sketch "Эскиз2" plane through (0, 0, 3) normal (0, 0, 1) x (1, 0, 0)
  point P0 (0, 0)
